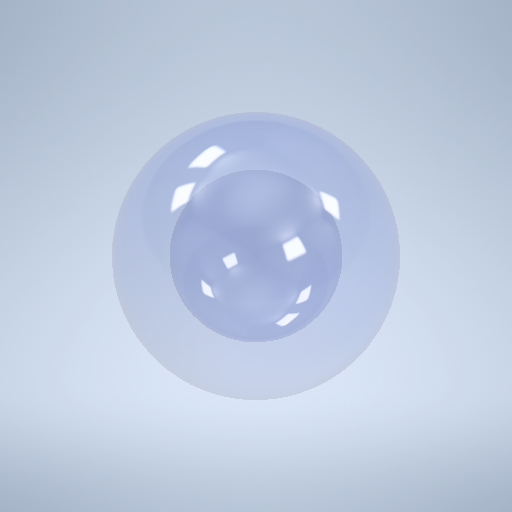
# Autodesk Inventor part: Esf_001
Saved by Autodesk Inventor 2025.2 (Build 292293000, 293)
## iProperties
Created: 2025-04-09
Part Number: Esf_001
Material: Vidro
Document SubType Name: Modeling
Designer: Formação
Density: 2.18 g/cm^3
Appearance: Azul tropical
Author: Formação
Autodesk Inventor part; units mm, degrees
ref_plane "YZ Plane" through (0, 0, 0) normal (1, 0, 0) x (0, 1, 0)
ref_plane "XZ Plane" through (0, 0, 0) normal (0, 1, 0) x (-1, 0, 0)
ref_plane "XY Plane" through (0, 0, 0) normal (0, 0, 1) x (1, 0, 0)
sketch "Esboço1" plane through (0, 0, 0) normal (0, 0, 1) x (1, 0, 0)
  line L0 (0, 7.5) -> (0, -7.5)
  arc A0 (0, 7.5) -> (0, -7.5) centre (0, 0) ccw
  arc A1 (0, 4.5) -> (0, -4.5) centre (0, 0) ccw
  point P0 (0, -4.5)
  dimension "d1" = 7.5
  dimension "d2" = 4.5
  constraints: 4 point on circle, 3 coincident, 2 centre point, 2 end point, 1 concentric, 1 midpoint, 1 point on line, 1 vertical
  measures "d1" radius of A0
  measures "d2" radius of A1
revolve "Revolução1" add sketch "Esboço1" angle 360 about axis through (0, 7.5, 0) along (0, -1, 0) contours L0 A1 A0
